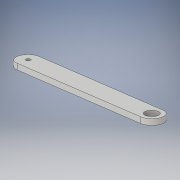
# Autodesk Inventor part: 連接4
Saved by Autodesk Inventor 2017 (Build 210142000, 142)
## iProperties
Part Number: 連接4
Material: 一般
Document SubType Name: Modeling
Designer: User
Density: 1 g/cm^3
Appearance: 預設
Author: User
Autodesk Inventor part; units mm, degrees
ref_plane "YZ Plane" through (0, 0, 0) normal (1, 0, 0) x (0, 1, 0)
ref_plane "XZ Plane" through (0, 0, 0) normal (0, 1, 0) x (-1, 0, 0)
ref_plane "XY Plane" through (0, 0, 0) normal (0, 0, 1) x (1, 0, 0)
sketch "草圖1" plane through (0, 0, 0) normal (0, 1, 0) x (-1, 0, 0)
  circle A0 centre (0, 0) radius 1.25
  line L0 (0, 0) -> (-80, 0)
  circle A1 centre (-80, 0) radius 3.6
  circle A2 centre (-80, 0) radius 6
  circle A3 centre (0, 0) radius 6
  line L1 (0, 6) -> (-80, 6)
  line L2 (-80, -6) -> (0, -6)
  dimension "d0" = 2.5
  dimension "d14" = 80
  dimension "d15" = 7.2
  dimension "d16" = 12
  dimension "d17" = 12
  constraints: 6 end point, 4 centre point, 4 coincident, 4 point on circle, 2 horizontal, 1 tangent
  measures "d0" diameter of A0
  measures "d14" distance of L0.start L0.end
  measures "d15" diameter of A1
  measures "d16" diameter of A2
  measures "d17" diameter of A3
extrude "擠出1" add sketch "草圖1" along normal mid plane 3
